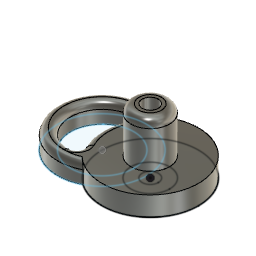
BikeBatteryTab v3 (Autodesk Fusion 360 design; units mm, degrees)
Autodesk Fusion 360 part; units mm, degrees
sketch "Sketch1" plane through (0, 0, 0) normal (0, 0, 1) x (1, 0, 0)
  circle A0 centre (0, 0) radius 3
  circle A1 centre (0, 0) radius 1.25
  circle A2 centre (0, 0) radius 7.5
  circle A3 centre (-7.5, 0.0183) radius 6.93
  circle A4 centre (-7.5, 0.0183) radius 4.9285
  dimension "d1" = 6
  dimension "d2" = 2.5
  dimension "d3" = 15
  constraint coincident A0.centre A1.centre
  constraint concentric A0 A1
  constraint coincident A2 A3.centre
  constraint concentric A3 A4
  measures "d1" diameter of A0
  measures "d2" diameter of A1
  measures "d3" diameter of A2
extrude "Extrude1" add sketch "Sketch1" along normal blind 10 contours A0 A1 A3 | A0 A1 A3 A4 | A0 A4
extrude "Extrude2" add sketch "Sketch1" along normal blind 3 contours A0 A2 A3 | A0 A2 A3 A4 | A0 A2 A3 A4 | A0 A2 A4 | A1 A3 | A1 A3
fillet "Fillet1" radius 1.25 1 edges at (-2.797, -1.0848, 10)
extrude "Extrude3" add sketch "Sketch1" along normal blind 3 contours A2 A3 A4
fillet "Fillet2" radius 1 2 edges at (-5.892, -4.6405, 1.5) (-5.8693, 4.6692, 1.5)
fillet "Fillet3" radius 1 4 edges at (-6.6744, 4.4673, 3) (-12.4284, 0.0303, 3) (-6.6961, -4.4347, 3) (-7.5, 0.0183, 3)
fillet "Fillet4" radius 1 1 edges at (-14.43, 0.0352, 3)
named bodies: "BikeBatteryCover"
